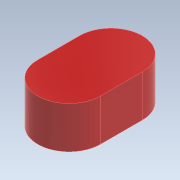
# Autodesk Inventor part: Passfeder16x8x8
Saved by Autodesk Inventor 2022 (Build 260153000, 153)
## iProperties
Created: 2022-03-11
Part Number: Passfeder16x8x8
Material: Generisch
Document SubType Name: Modeling
Designer: 123St
Density: 1 g/cm^3
Appearance: Rot
Mass: 1.67278 g
Surface Area: 8.47788 cm^2
Volume: 1.67278 cm^3
Passfeder_length: 20,000 mm
Passfeder_height: 8,000 mm
Passfeder_width: 12,000 mm
Author: 123St
Autodesk Inventor part; units mm, degrees
ref_plane "YZ Plane" through (0, 0, 0) normal (1, 0, 0) x (0, 1, 0)
ref_plane "XZ Plane" through (0, 0, 0) normal (0, 1, 0) x (-1, 0, 0)
ref_plane "XY Plane" through (0, 0, 0) normal (0, 0, 1) x (1, 0, 0)
sketch "Skizze1" plane through (0, 0, 0) normal (0, 1, 0) x (-1, 0, 0)
  line L0 (0, 4) -> (0, -4) construction
  line L1 (-6, 4) -> (-6, -4)
  line L2 (6, -4) -> (6, 4)
  arc A0 (6, 4) -> (-6, 4) centre (0, 4) ccw
  arc A1 (-6, -4) -> (6, -4) centre (0, -4) ccw
  line L3 (0, -12.6) -> (0, 12.6) construction
  point P0 (0, 0)
  point P1 (0, 0)
  point P2 (0, 10)
  point P3 (0, -10)
  dimension "d1" = 12
  dimension "d4" = 20
  constraints: 8 end point, 6 point on circle, 4 tangent, 2 centre point, 2 point on line, 1 coincident, 1 collinear, 1 midpoint, 1 parallel, 1 vertical
  measures "d1" distance between parallel lines of L1 L2
  measures "d4" distance of point (0, -10) point (0, 10)
extrude "Extrusion1" add sketch "Skizze1" along normal blind 8
equation "\"d1\" = Passfeder_width"
equation "\"d4\" = Passfeder_length"
equation "\"d2\" = Passfeder_height"
equation "\"Passfeder_height\" = 8"
equation "\"Passfeder_width\" = 12"
equation "\"Passfeder_length\" = 20"
